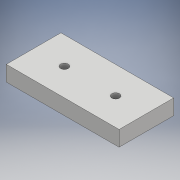
# Autodesk Inventor part: LearnbotUnion
Saved by Autodesk Inventor 2017 (Build 210142000, 142)
## iProperties
Part Number: LearnbotUnion
Material: Genérico
Document SubType Name: Modeling
Designer: Roberto
Density: 1 g/cm^3
Appearance: Valor por defecto
Author: Roberto
Autodesk Inventor part; units mm, degrees
ref_plane "YZ Plane" through (0, 0, 0) normal (1, 0, 0) x (0, 1, 0)
ref_plane "XZ Plane" through (0, 0, 0) normal (0, 1, 0) x (-1, 0, 0)
ref_plane "XY Plane" through (0, 0, 0) normal (0, 0, 1) x (1, 0, 0)
sketch "Boceto1" plane through (0, 0, 0) normal (0, 0, 1) x (1, 0, 0)
  line L0 (0.1, 1.065) -> (1.1, 1.065)
  line L1 (1.1, 1.065) -> (1.1, 0)
  circle A0 centre (0.5, 0.5325) radius 0.075
  line L2 (0.1, 0) -> (7.6, 0)
  line L3 (0, 1.8248) -> (0, 0)
  line L4 (0, 1.065) -> (0.1, 1.065)
  line L5 (0.1, 0) -> (0, 0)
  line L6 (-0.1, 1.065) -> (-1.1, 1.065)
  line L7 (-1.1, 1.065) -> (-1.1, 0)
  circle A1 centre (-0.5, 0.5325) radius 0.075
  line L8 (-0.1, 0) -> (-7.6, 0)
  line L9 (0, 1.065) -> (-0.1, 1.065)
  line L10 (-0.1, 0) -> (0, 0)
  point P0 (0, 0)
  constraints: 22 end point, 6 symmetric about line, 2 centre point, 1 other
extrude "Extrusión1" add sketch "Boceto1" along normal blind 0.3
